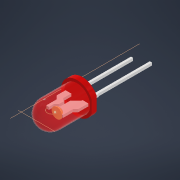
# Autodesk Inventor part: LED 5mm
Saved by Autodesk Inventor 2022 (Build 260153000, 153)
## iProperties
Created: 2022-10-04
Part Number: LED 5mm
Material: Generic
Document SubType Name: Modeling
Designer: ipien
Density: 1 g/cm^3
Appearance: Default
Author: ipien
Autodesk Inventor part; units mm, degrees
ref_plane "YZ Plane" through (0, 0, 0) normal (1, 0, 0) x (0, 1, 0)
ref_plane "XZ Plane" through (0, 0, 0) normal (0, 1, 0) x (-1, 0, 0)
ref_plane "XY Plane" through (0, 0, 0) normal (0, 0, 1) x (1, 0, 0)
sketch "Sketch1" plane through (0, 0, 0) normal (0, 1, 0) x (-1, 0, 0)
  line L0 (-1.93, -19.18) -> (-1.53, -19.18)
  line L1 (-4.47, -20.18) -> (-4.07, -20.18)
  line L2 (-0.5, -2.5) -> (-5.5, -2.5) construction
  line L3 (-5.5, -2.5) -> (-5.5, -7.5)
  line L4 (-5.5, -7.5) -> (-0.5, -7.5)
  line L5 (-0.5, -7.5) -> (-0.5, -2.5)
  line L6 (0, -7.5) -> (-6, -7.5)
  line L7 (-6, -7.5) -> (-6, -8.5)
  line L8 (-6, -8.5) -> (0, -8.5)
  line L9 (0, -8.5) -> (0, -7.5)
  arc A0 (-0.5, -2.5) -> (-5.5, -2.5) centre (-3, -2.5) ccw
  line L10 (0, -24.216) -> (0, 4.0361) projected
  line L11 (17.1925, 0) -> (-9.8654, 0) projected
  line L12 (-3, -8.5) -> (-3, -19.8408) construction
  line L13 (-1.53, -19.18) -> (-1.53, -10)
  line L14 (-1.93, -19.18) -> (-1.93, -10)
  line L15 (-4.07, -20.18) -> (-4.07, -10)
  line L16 (-4.47, -20.18) -> (-4.47, -10)
  line L17 (-3, -8.5) -> (-3, 0)
  line L18 (-6, -19.8408) -> (0, -19.8408) construction
  line L19 (-1.43, -9) -> (-1.53, -9)
  line L20 (-2.03, -9) -> (-2.03, -10)
  line L21 (-2.03, -10) -> (-1.93, -10)
  line L22 (-1.43, -10) -> (-1.43, -9)
  line L23 (-3.97, -9) -> (-4.07, -9)
  line L24 (-4.57, -9) -> (-4.57, -10)
  line L25 (-4.57, -10) -> (-4.47, -10)
  line L26 (-3.97, -10) -> (-3.97, -9)
  line L27 (-1.93, -9) -> (-2.03, -9)
  line L28 (-4.07, -9) -> (-4.07, -7.25)
  line L29 (-4.47, -9) -> (-4.57, -9)
  line L30 (-4.07, -10) -> (-3.97, -10)
  line L31 (-1.53, -10) -> (-1.43, -10)
  line L32 (-4.47, -9) -> (-4.47, -8.18)
  line L33 (-1.93, -9) -> (-1.93, -5.9716)
  line L34 (-1.53, -9) -> (-1.53, -8.18)
  line L35 (-4.47, -8.18) -> (-5.15, -7.5)
  line L36 (-1.53, -8.18) -> (-0.85, -7.5)
  line L37 (-0.85, -7.5) -> (-0.85, -5.85)
  line L38 (-5.15, -7.5) -> (-5.15, -5.5986)
  line L39 (-5.15, -5.5986) -> (-4.65, -5.0986)
  line L40 (-4.65, -5.0986) -> (-4.65, -3.1972)
  line L41 (-4.65, -3.1972) -> (-2.5028, -3.1972)
  line L42 (-0.85, -5.85) -> (-1.5028, -5.1972)
  line L43 (-1.5028, -5.1972) -> (-1.5028, -3.1972)
  line L44 (-1.5028, -3.1972) -> (-2.0028, -3.1972)
  line L45 (-2.0028, -3.1972) -> (-2.0028, -4.1043)
  line L46 (-2.0028, -4.1043) -> (-2.5, -4.6016)
  line L47 (-2.5, -4.6016) -> (-2.5, -5.6016)
  line L48 (-2.5, -5.6016) -> (-2.3, -5.6016)
  line L49 (-2.3, -5.6016) -> (-1.93, -5.9716)
  line L50 (8.8309, -12.5892) -> (8.8309, -17.0713)
  line L51 (8.7309, -12.5892) -> (8.8309, -12.5892)
  line L52 (8.8309, -17.0713) -> (9.3309, -17.0713)
  line L53 (9.3309, -17.0713) -> (9.3309, -12.5892)
  line L54 (11.3309, -18.2444) -> (11.8309, -18.2444)
  line L55 (11.3309, -12.5815) -> (11.3309, -18.2444)
  line L56 (11.8309, -18.2444) -> (11.8309, -12.5815)
  line L57 (8.2266, -6.0537) -> (8.2266, -7.4999)
  line L58 (8.5861, -5.6941) -> (8.2266, -6.0537)
  line L59 (8.5861, -4.3452) -> (8.5861, -5.6941)
  line L60 (8.2266, -7.4999) -> (8.8309, -8.1043)
  line L61 (9.3309, -7.3282) -> (9.7365, -6.9226)
  line L62 (9.7365, -6.9226) -> (10.3309, -6.9226)
  line L63 (10.3309, -6.9226) -> (10.3309, -5.844)
  line L64 (8.5861, -4.3452) -> (11.2106, -4.3452)
  line L65 (10.8309, -6.0512) -> (10.8309, -6.9149)
  line L66 (10.8309, -6.9149) -> (11.1527, -6.9149)
  line L67 (11.2393, -4.3452) -> (11.2106, -4.3452)
  line L68 (11.1527, -6.9149) -> (11.3309, -7.0932)
  line L69 (11.8309, -8.0966) -> (12.4276, -7.4999)
  line L70 (12.4276, -7.4999) -> (12.4276, -5.8553)
  line L71 (9.4309, -11.5892) -> (9.3309, -11.5892)
  line L72 (11.8309, -11.5815) -> (11.8309, -8.0966)
  line L73 (8.8309, -8.1043) -> (8.8309, -11.5892)
  line L74 (11.3309, -7.0932) -> (11.3309, -11.5815)
  line L75 (9.3309, -11.5892) -> (9.3309, -7.3282)
  line L76 (10.3309, -5.844) -> (11.2106, -4.9643)
  line L77 (11.7107, -5.1714) -> (10.8309, -6.0512)
  line L78 (11.2106, -4.3452) -> (11.2393, -4.3452) construction
  line L79 (12.4276, -5.8553) -> (12.2082, -5.6359)
  line L80 (11.2106, -4.2719) -> (11.2106, -4.3452)
  line L81 (11.2106, -4.9643) -> (11.2106, -4.2719)
  line L82 (11.2106, -4.2719) -> (11.2393, -4.3452)
  line L83 (11.7107, -4.3453) -> (11.7107, -5.1714)
  line L84 (10.8445, -3.7709) -> (11.3445, -3.7709) construction
  spline S0 degree 3 poles (11.9954, -4.3997) (11.9862, -4.3486) (11.9578, -4.2521) (11.8889, -4.1254) (11.7974, -4.0171) (11.6749, -3.9177) (11.5186, -3.8358) (11.3301, -3.782) (11.1322, -3.7647) (10.9338, -3.7851) (10.7437, -3.8443) (10.5851, -3.9352) (10.4598, -4.0478) (10.3654, -4.1727) (10.2931, -4.3216) (10.262, -4.4371) (10.2513, -4.4991) knots 0 0 0 0 0.0625 0.125 0.1875 0.25 0.333333 0.416667 0.5 0.583333 0.666667 0.75 0.8125 0.875 0.9375 1 1 1 1
  line L85 (12.2082, -4.3453) -> (11.7107, -4.3453)
  line L86 (12.2082, -5.6359) -> (12.2082, -4.3453)
  line L87 (9.3309, -12.5892) -> (9.4309, -12.5892)
  line L88 (11.2309, -12.5815) -> (11.3309, -12.5815)
  line L89 (11.8309, -12.5815) -> (11.9309, -12.5815)
  line L90 (8.7309, -11.5892) -> (8.7309, -12.5892)
  line L91 (8.8309, -11.5892) -> (8.7309, -11.5892)
  line L92 (9.4309, -12.5892) -> (9.4309, -11.5892)
  line L93 (11.3309, -11.5815) -> (11.2309, -11.5815)
  line L94 (11.2309, -11.5815) -> (11.2309, -12.5815)
  line L95 (11.9309, -12.5815) -> (11.9309, -11.5815)
  line L96 (11.9309, -11.5815) -> (11.8309, -11.5815)
  line L97 (13.3271, -7.4999) -> (7.3271, -7.4999)
  line L98 (7.3271, -7.4999) -> (7.3271, -8.4999)
  line L99 (7.3271, -8.4999) -> (13.3271, -8.4999)
  line L100 (13.3271, -8.4999) -> (13.3271, -7.4999)
  line L101 (12.4276, -7.4999) -> (8.2266, -7.4999)
  line L102 (12.8271, -7.4999) -> (7.8271, -7.4999)
  line L103 (7.8271, -7.4999) -> (7.8271, -2.4999)
  line L104 (7.8271, -2.4999) -> (12.8271, -2.4999) construction
  line L105 (12.8271, -2.4999) -> (12.8271, -7.4999)
  arc A1 (12.8271, -2.4999) -> (7.8271, -2.4999) centre (10.3271, -2.4999) ccw
  line L106 (-2.5028, -3.1972) -> (-2.5028, -3.8972)
  line L107 (-2.5028, -3.8972) -> (-3, -4.3944)
  line L108 (-3, -4.3944) -> (-3, -5.9975)
  line L109 (-3, -6.18) -> (-4.07, -7.25)
  line L110 (-2.5028, -3.1972) -> (-2.0028, -3.1972) construction
  line L111 (-2.5, -5.6016) -> (-3, -5.9975) construction
  point P0 (0, 0)
  point P1 (-3, -7.5)
  point P2 (0, -8)
  point P3 (-1.73, -19.18)
  point P4 (-4.27, -20.18)
  point P5 (-3, -7.5)
  point P6 (0, 0)
  point P7 (7.8271, -7.4999)
  point P8 (10.3271, -7.4999)
  point P9 (-3, -5.196)
  point P10 (-3, -4.3944)
  point P11 (-3, -3.1972)
  dimension "d10" = 5
  dimension "d12" = 6
  dimension "d13" = 5
  dimension "d14" = 6
  dimension "Jarak_Kaki" = 2.54
  dimension "d18" = 1
  dimension "d19" = 0.4
  dimension "d20" = 1.27
  dimension "Panjang_Kaki" = 12
  dimension "d30" = 0.6
  dimension "d31" = 1
  dimension "d32" = 0.5
  dimension "d34" = 135
  dimension "d35" = 0.35
  dimension "d51" = 0.5
  dimension "d76" = 1.65
  dimension "d82" = 2.5
  dimension "d83" = 0.5
  dimension "d84" = 0.5
  dimension "d85" = 1
  dimension "d86" = 0.5
  dimension "d87" = 0.5
  dimension "d89" = 0.7
  dimension "d92" = 0.5
  dimension "d93" = 0.25
  dimension "d95" = 1
  dimension "d104" = 0.2
  dimension "d106" = 2
  constraints: 218 end point, 25 parallel, 16 vertical, 15 equal length, 13 perpendicular, 13 point on line, 12 midpoint, 10 horizontal, 5 point on circle, 2 centre point, 1 collinear, 1 tangent, 5 other
  measures "d10" distance of L2.end L3.end
  measures "d12" distance of L7.end L8.end
  measures "d13" distance between parallel lines of L3 L5
  measures "d14" distance between parallel lines of L8 L2
  measures "Jarak_Kaki" horizontal distance of point (-4.27, -20.18) point (-1.73, -19.18)
  measures "d18" distance between parallel lines of L1 L0
  measures "d19" distance of L0.start L0.end
  measures "d20" distance from line of point (-1.73, -19.18) L12
  measures "Panjang_Kaki" distance of L1.start L32.end
  measures "d30" distance between parallel lines of L22 L20
  measures "d31" distance of L22.start L19.start
  measures "d32" distance between parallel lines of L19 L8
  measures "d34" angle of L32 L35
  measures "d35" distance from line of L3 L35.end
  measures "d51" horizontal distance of L38.end L39.end
  measures "d76" distance of L36.end L37.end
  measures "d82" radius of A1
  measures "d83" distance of L97.start L102.start
  measures "d84" distance of L97.end L102.end
  measures "d85" distance of L99.end L97.start
  measures "d86" distance between parallel lines of L106 L45
  measures "d87" distance between parallel lines of L46 L107
  measures "d89" distance of L106.end L41.end
  measures "d92" distance of L43.end L44.end
  measures "d93" distance from line of L4 L28.end
  measures "d95" distance of L46.end L47.end
  measures "d104" distance of L47.end L48.end
  measures "d106" distance of L42.end L43.end
revolve "Revolution1" add sketch "Sketch1" angle 360 about axis through (3, 0, -8.5) along (0, 0, 1) contours L33 L49 L48 L47 L46 L45 L44 L43 L42 L37 L4 | L4 L17 L107 L106 L41 A0 L5 L37 L42 L43 L44 L45 L46 L47 L48 L49 L33 | L17 L41 L106 L107
shell "Shell1" thickness 0.1 removed faces 1 at (3.6238, -0.5526, -7.5)
revolve "Revolution2" add sketch "Sketch1" angle 360 about axis through (3, 0, -8.5) along (0, 0, 1) separate body contours L33 L4 L36 L34 L8 | L8 L17 L4 L33 | L34 L36 L4 L6 L9 L8
sketch "Sketch2" plane through (3, 0, -7.5) normal (0, 0, 1) x (1, 0, 0)
  line L0 (2.75, 2.5) -> (3.75, 2.5)
  line L1 (3.75, 2.5) -> (3.75, -2.5)
  line L2 (3.75, -2.5) -> (2.75, -2.5)
  line L3 (2.75, -2.5) -> (2.75, 2.5)
  circle A0 centre (0, 0) radius 2.5 projected
  circle A1 centre (0, 0) radius 2.5 projected
  line L4 (-3, -4.2) -> (-3, 4.2) construction
  line L5 (2.5, -1.6681) -> (2.5, 1.3873) construction
  line L6 (-4.368, 0) -> (5.2078, 0) projected
  point P0 (-3, 0)
  point P1 (2.75, 0)
  dimension "d110" = 0.25
  dimension "d111" = 5
  dimension "d112" = 1
  constraints: 10 end point, 3 parallel, 1 horizontal, 1 midpoint, 1 perpendicular, 1 point on line, 1 tangent, 1 vertical
  measures "d110" distance between parallel lines of L5 L3
  measures "d111" distance of L0.end L1.end
  measures "d112" distance of L0.start L0.end
extrude "Extrusion1" cut sketch "Sketch2" against normal up to next contours L0 L1 L6 L3 | L6 L1 L2 L3 bodies 2
extrude "Extrusion2" add sketch "Sketch1" along normal mid plane 0.5 separate body contours L14 L21 L20 L27 L33 L8 L34 L19 L22 L31 L13 L0 | L33 L4 L36 L34 L8 | L33 L49 L48 L47 L46 L45 L44 L43 L42 L37 L4 | L28 L23 L26 L30 L15 L1 L16 L25 L24 L29 L32 L8 | L8 L32 L35 L4 L28 | L4 L38 L39 L40 L41 L17 L109 L28 | L17 L41 L106 L107
sketch "Sketch3" plane through (2.4, 0, -4) normal (0, 1, 0) x (1, 0, 0)
  line L0 (0.1028, -0.1028) -> (0.1028, -0.8028) projected
  line L1 (0.1028, -0.8028) -> (0.1694, -0.2824) construction
  line L2 (0.1694, -0.2824) -> (0.7748, -0.0028) construction
  line L3 (0.7748, -0.0028) -> (1.0028, -0.0028) construction
  spline S0 degree 3 poles (0.1028, -0.8028) (0.1694, -0.2824) (0.7748, -0.0028) (1.0028, -0.0028) knots 1 1 1 1 2 2 2 2
  line L4 (0.1028, -0.8028) -> (2.25, -0.8028) projected
  line L5 (1.0028, -0.0028) -> (1.1028, -0.0028)
  line L6 (1.1028, -0.0028) -> (1.1028, -0.8028)
  dimension "d99" = 0.8
  dimension "d100" = 0.9
  dimension "d101" = 0.1
  constraints: 4 end point, 2 horizontal, 1 perpendicular, 1 point on line, 3 other
  measures "d99" distance from line of L4 L3.end
  measures "d101" distance of L3.end L5.end
revolve "Revolution3" cut sketch "Sketch3" angle 360 about axis through (3.5028, 0, -3.9972) along (0, 0, 1) bodies 3
revolve "Revolution4" add sketch "Sketch3" angle 360 about axis through (3.5028, 0, -3.9972) along (0, 0, 1) separate body
sketch "Sketch4" plane through (3.5028, 0, -3.1972) normal (0, 0, 1) x (1, 0, 0)
  circle A0 centre (-1.7728, 0) radius 0.05
  line L0 (-2, -0.25) -> (-2, 0.25) construction
  line L1 (-2, 0.25) -> (-1.5, 0.25) construction
  line L2 (-1.5728, 0.25) -> (-1.9728, 0.25) construction
  line L3 (-2, 0) -> (-1.7728, 0) construction
  line L4 (-1.7728, 0) -> (-1.7728, 0.25) construction
  line L5 (-1.7728, 0.25) -> (-2, 0.25) construction
  line L6 (-2, 0.25) -> (-2, 0) construction
  circle A1 centre (0, 0) radius 0.05
  point P0 (-3.5028, 0)
  dimension "d109" = 0.1
  constraints: 12 end point, 2 centre point, 2 coincident, 2 midpoint, 2 parallel, 1 collinear, 1 equal radius, 1 horizontal, 1 perpendicular, 1 vertical
  measures "d109" diameter of A0
sketch "Sketch5" plane through (0, 0, 0) normal (0, 1, 0) x (-1, 0, 0)
  line L0 (-5.5, -2.5) -> (-0.5, -2.5) construction
  line L1 (-5.5, -7.5) -> (-0.5, -7.5) construction
  line L2 (-1.5028, -3.1972) -> (-2.0028, -3.1972) construction
  line L3 (-4.5028, -3.1972) -> (-2.5028, -3.1972) construction
  line L4 (-1.7528, -3.1972) -> (-3.5028, -3.1972) construction
  arc A0 (-1.7528, -3.1972) -> (-3.5028, -3.1972) centre (-2.6278, -3.1972) ccw
  point P0 (0, 0)
  constraints: 3 midpoint, 2 end point, 2 point on circle, 1 centre point
sweep "Sweep1" add profiles "Sketch4" path "Sketch5" separate body contours A0
equation "\"d10\" = Diameter_Led"
equation "\"d13\" = Diameter_Led"
equation "\"d20\" = 0.5 * Jarak_Kaki"
equation "\"Diameter_Led\" = 5"
body "Solid1"
body "Solid2"
body "Solid3"
body "Solid4"
body "Solid5"
